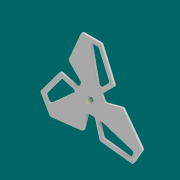
# Autodesk Inventor part: BatteryCoverLid
Saved by Autodesk Inventor 2020.4 (Build 244396010, 396A)
## iProperties
Created: 2022-09-11
Part Number: BatteryCoverLid
Material: Generic
Document SubType Name: Sheet Metal
Designer: Val
Density: 1 g/cm^3
Sheet Metal Rule: Default
Appearance: Default
Author: Val
Autodesk Inventor part; units mm, degrees
ref_plane "YZ Plane" through (0, 0, 0) normal (1, 0, 0) x (0, 1, 0)
ref_plane "XZ Plane" through (0, 0, 0) normal (0, 1, 0) x (-1, 0, 0)
ref_plane "XY Plane" through (0, 0, 0) normal (0, 0, 1) x (1, 0, 0)
sketch "Sketch1" plane through (0, 0, 0) normal (0, 0, 1) x (1, 0, 0)
  line L0 (15.875, 15.875) -> (-15.875, 15.875)
  line L1 (-15.875, 15.875) -> (-21.6857, 5.8107)
  line L2 (-21.6857, 5.8107) -> (-5.8107, -21.6857)
  line L3 (-5.8107, -21.6857) -> (5.8107, -21.6857)
  line L4 (5.8107, -21.6857) -> (21.6857, 5.8107)
  line L5 (21.6857, 5.8107) -> (15.875, 15.875)
  line L6 (50.6335, 13.5672) -> (21.6857, 5.8107)
  line L7 (37.0663, 37.0663) -> (15.875, 86.1801)
  line L8 (-15.875, 86.1801) -> (15.875, 86.1801)
  line L9 (-15.875, 86.1801) -> (-37.0663, 37.0663)
  line L10 (-37.0663, 37.0663) -> (-15.875, 15.875)
  line L11 (15.875, 15.875) -> (37.0663, 37.0663)
  line L12 (82.5716, -29.3419) -> (50.6335, 13.5672)
  line L13 (82.5716, -29.3419) -> (66.6966, -56.8382)
  line L14 (13.5672, -50.6335) -> (66.6966, -56.8382)
  line L15 (5.8107, -21.6857) -> (13.5672, -50.6335)
  line L16 (-13.5672, -50.6335) -> (-5.8107, -21.6857)
  line L17 (-66.6966, -56.8382) -> (-13.5672, -50.6335)
  line L18 (-66.6966, -56.8382) -> (-82.5716, -29.3419)
  line L19 (-50.6335, 13.5672) -> (-82.5716, -29.3419)
  line L20 (-21.6857, 5.8107) -> (-50.6335, 13.5672)
  circle A0 centre (0, 0) radius 3.675
  dimension "d0" = 7.35
  dimension "d1" = 113.339
  dimension "d2" = 111.661
  dimension "d3" = 166.678
  dimension "d4" = 6.661
  dimension "d5" = 81.661
  dimension "d6" = 46.678
  dimension "d7" = 126.661
  dimension "d8" = 51.661
  dimension "d9" = 60
  dimension "d10" = 73.322
  dimension "d11" = 60
  dimension "d12" = 70.305
  dimension "d13" = 107.8657
  dimension "d14" = 37.5607
  dimension "d15" = 107.8657
  dimension "d16" = 37.5607
  dimension "d17" = 70.305
  dimension "d18" = 48.7179
  dimension "d19" = 86.18
  dimension "d20" = 0
  dimension "d21" = 48.7179
  dimension "d22" = 0
  dimension "d23" = 48.7179
  dimension "d24" = 48.7179
  dimension "d25" = 48.7179
  dimension "d26" = 48.7179
  dimension "d27" = 48.7179
  dimension "d28" = 86.18
  measures "d0" diameter of A0
  measures "d1" angle of L12 L13
  measures "d2" angle of L12 L6
  measures "d3" angle of L12 L7
  measures "d4" angle of L12 L5
  measures "d5" angle of L12 L11
  measures "d6" angle of L12 L14
  measures "d7" angle of L12 L0
  measures "d8" angle of L12 L16
  measures "d9" angle of L12 L9
  measures "d10" angle of L12 L19
  measures "d11" angle of L12 L17
  measures "d12" distance between parallel lines of L13 L4
  measures "d13" distance between parallel lines of L13 L1
  measures "d14" distance between parallel lines of L5 L2
  measures "d15" distance between parallel lines of L18 L5
  measures "d16" distance between parallel lines of L0 L3
  measures "d17" distance between parallel lines of L8 L0
  measures "d18" distance from line of point (0, 0) L12
  measures "d19" distance from line of point (0, 0) L13
  measures "d20" distance from line of point (0, 0) L6
  measures "d21" distance from line of point (0, 0) L7
  measures "d22" distance from line of point (0, 0) L11
  measures "d23" distance from line of point (0, 0) L14
  measures "d24" distance from line of point (0, 0) L9
  measures "d25" distance from line of point (0, 0) L19
  measures "d26" distance from line of point (0, 0) L17
  measures "d27" distance from line of point (0, 0) L12
  measures "d28" distance from line of point (0, 0) L13
extrude "Plate1" add sketch "Sketch1" along normal blind 2.54
fillet "Corner Round1" radius 3.175 18 edges at (-15.875, 86.1801, 1.27) (15.875, 86.1801, 1.27) (-37.0663, 37.0663, 1.27) (-15.875, 15.875, 1.27) (37.0663, 37.0663, 1.27) (15.875, 15.875, 1.27) (21.6857, 5.8107, 1.27) (50.6335, 13.5672, 1.27) (82.5716, -29.3419, 1.27) (66.6966, -56.8382, 1.27) (13.5672, -50.6335, 1.27) (5.8107, -21.6857, 1.27) (-5.8107, -21.6857, 1.27) (-13.5672, -50.6335, 1.27) (-66.6966, -56.8382, 1.27) (-82.5716, -29.3419, 1.27) (-50.6335, 13.5672, 1.27) (-21.6857, 5.8107, 1.27)
sketch "Sketch2" plane through (0, 0, 0) normal (0, 0, -1) x (-1, 0, 0)
  line L0 (1.001, 79.8301) -> (-11.699, 79.8301)
  line L1 (-11.699, 79.8301) -> (-29.5281, 38.5084)
  line L2 (-29.5281, 38.5084) -> (-11.5942, 20.5744)
  line L3 (-11.5942, 20.5744) -> (1.001, 79.8301)
  line L4 (-13.787, 86.1801) -> (13.787, 86.1801) projected
  line L5 (-17.5977, 17.5977) -> (-35.5423, 35.5423) projected
  line L6 (-36.2124, 39.0452) -> (-16.7022, 84.2629) projected
  arc A0 (-36.2124, 39.0452) -> (-35.5423, 35.5423) centre (-33.2972, 37.7873) ccw projected
  line L7 (48.1133, 6.3179) -> (74.9843, -29.7834)
  line L8 (81.3249, -27.6669) -> (51.9203, 11.8383) projected
  line L9 (74.9843, -29.7834) -> (68.6343, -40.7819)
  line L10 (68.6343, -40.7819) -> (23.615, -0.2464)
  line L11 (23.615, -0.2464) -> (48.1133, 6.3179)
  line L12 (-12.0209, -20.328) -> (-18.5852, -44.8263)
  line L13 (-18.5852, -44.8263) -> (-63.2854, -50.0466)
  line L14 (-63.2854, -50.0466) -> (-69.6354, -39.0481)
  line L15 (-69.6354, -39.0481) -> (-12.0209, -20.328)
  line L16 (24.0389, 6.4412) -> (48.5516, 13.0094) projected
  line L17 (81.5276, -31.1501) -> (67.7406, -55.0299) projected
  line L18 (-6.4412, -24.0389) -> (-13.0094, -48.5516) projected
  line L19 (-15.7079, -50.8835) -> (-64.6227, -56.596) projected
  line L20 (-67.7406, -55.0299) -> (-81.5276, -31.1501) projected
  point P0 (0, 0)
  dimension "d31" = 6.35
  dimension "d32" = 6.35
  dimension "d33" = 6.35
  dimension "d36" = 6.35
  dimension "d37" = 6.35
  dimension "d38" = 6.35
  dimension "d39" = 6.35
  dimension "d40" = 6.35
  dimension "d41" = 6.35
  dimension "d42" = 57
  dimension "d43" = 57
  dimension "d44" = 57
  dimension "d45" = 12.7
  constraints: 24 end point, 9 parallel, 2 equal length, 1 horizontal
  measures "d31" distance between parallel lines of L4 L0
  measures "d32" distance between parallel lines of L5 L2
  measures "d33" distance between parallel lines of L6 L1
  measures "d36" distance between parallel lines of L8 L7
  measures "d37" distance between parallel lines of L17 L9
  measures "d38" distance between parallel lines of L16 L11
  measures "d39" distance between parallel lines of L18 L12
  measures "d40" distance between parallel lines of L19 L13
  measures "d41" distance between parallel lines of L20 L14
  measures "d42" angle of L12 L15
  measures "d43" angle of L3 L2
  measures "d44" angle of L10 L11
  measures "d45" distance of L7.end L9.end
extrude "Cut1" cut sketch "Sketch2" against normal blind 2.54
fillet "Corner Round2" radius 3.175 12 edges at (-23.615, -0.2464, 1.27) (-48.1133, 6.3179, 1.27) (-74.9843, -29.7834, 1.27) (-68.6343, -40.7819, 1.27) (-1.001, 79.8301, 1.27) (11.699, 79.8301, 1.27) (29.5281, 38.5084, 1.27) (11.5942, 20.5744, 1.27) (12.0209, -20.328, 1.27) (18.5852, -44.8263, 1.27) (69.6354, -39.0481, 1.27) (63.2854, -50.0466, 1.27)
equation "\"d32\" = d31"
equation "\"d33\" = d31"
equation "\"d36\" = d31"
equation "\"d37\" = d31"
equation "\"d38\" = d31"
equation "\"d39\" = d31"
equation "\"d40\" = d31"
equation "\"d41\" = d31"
equation "\"d46\" = Thickness"
equation "\"d29\" = Thickness"
equation "\"BendRadius\" = Thickness"
equation "\"BendReliefWidth\" = Thickness"
equation "\"BendReliefDepth\" = 0.5 * Thickness"
equation "\"CornerReliefSize\" = 4 * Thickness"
equation "\"MinimumRemnant\" = 2 * Thickness"
equation "\"TransitionRadius\" = BendRadius"
equation "\"JacobiRadiusSize\" = BendRadius"
equation "\"GapSize\" = Thickness"
equation "\"Thickness\" = 2.54"
body "Solid1"
